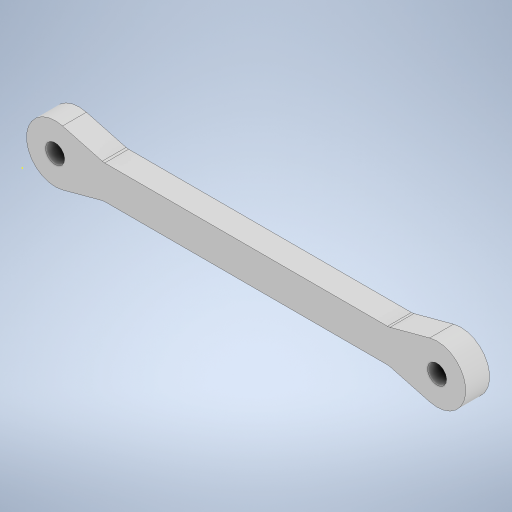
# Autodesk Inventor part: STEP translator 7.5 1
Saved by Autodesk Inventor 2023 (Build 270158000, 158)
## iProperties
Created: 2023-11-09
Part Number: STEP translator 7.5 1
Material: Genérico
Description: Model
Document SubType Name: Modeling
Designer: JULIAN
Authority: Unknown
Density: 1 g/cm^3
Appearance: Valor por defecto
Title: Shape Model
Autodesk Inventor part; units mm, degrees
ref_plane "YZ Plane" through (0, 0, 0) normal (1, 0, 0) x (0, 1, 0)
ref_plane "XZ Plane" through (0, 0, 0) normal (0, 1, 0) x (-1, 0, 0)
ref_plane "Plano de trabajo1" through (86.86, 8.06, 0.025) normal (0, 0, -1) x (-0.9876, 0.157, 0)
sketch "Boceto1" plane through (86.86, 8.06, 0.025) normal (0, 0, -1) x (-0.9876, 0.157, 0)
  line L0 (0.3099, -7.9427) -> (0.3097, -7.9404)
  circle A0 centre (-0.3141, -1.974) radius 1.9997
  arc A1 (2.1306, 3.5042) -> (0.3097, -7.9404) centre (-0.3141, -1.974) ccw
  arc A2 (76.2508, -20.0134) -> (78.0703, -8.566) centre (78.6942, -14.5335) ccw
  circle A3 centre (78.6942, -14.5335) radius 2
  line L1 (10.4901, -0.1486) -> (9.9896, 0)
  line L2 (69.5109, -9.4609) -> (68.989, -9.4469)
  line L3 (67.8902, -16.3602) -> (68.3907, -16.5087)
  line L4 (9.3912, -7.0618) -> (8.8693, -7.0478)
  line L5 (9.9896, 0) -> (2.1306, 3.5042)
  line L6 (8.8693, -7.0478) -> (0.3097, -7.9404)
  line L7 (9.3912, -7.0618) -> (67.8902, -16.3602)
  line L8 (68.3907, -16.5087) -> (76.2508, -20.0134)
  line L9 (78.0703, -8.566) -> (69.5109, -9.4609)
  line L10 (68.989, -9.4469) -> (10.4901, -0.1486)
  point P0 (84.5179, -21.5953)
  point P1 (2.1295, 3.5047)
  point P2 (78.0703, -8.566)
  point P3 (1.5536, -1.2595)
  point P4 (76.719, -14.2196)
  constraints: 22 end point, 6 point on circle, 2 centre point, 2 coincident, 2 parallel, 6 other
extrude "Extrusión1" add sketch "Boceto1" along normal blind 5
sketch "Boceto2" plane through (86.86, 8.06, 0.025) normal (0, 0, 1) x (0.9876, -0.157, 0)
  point P0 (-84.5179, -21.5953)
